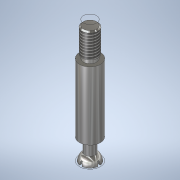
# Autodesk Inventor part: Connecting Pin L24
Saved by Autodesk Inventor 2022 (Build 260153000, 153)
## iProperties
Perskaiciuoti: 1
RuleStatus: InUse
Created: 2009-08-21
Material: Nickel-Copper Alloy 400
Description: Minifix Connecting Pin
Document SubType Name: Modeling
Designer: Saulius Dereskeviciu
Mass: 10.9743 g
Surface Area: 8.70491 cm^2
Volume: 1.24284 cm^3
Density: 8.83 g/cm^3
Appearance: Chrome - Polished
Author: Saulius Dereskeviciu
Part Number: Connecting Pin L24
Autodesk Inventor part; units mm, degrees
ref_plane "YZ Plane" through (0, 0, 0) normal (1, 0, 0) x (0, 1, 0)
ref_plane "XZ Plane" through (0, 0, 0) normal (0, 1, 0) x (-1, 0, 0)
sketch "Sketch1" plane through (0, 0, 0) normal (0, 0, 1) x (1, 0, 0)
  circle A0 centre (0, 0) radius 2
  dimension "d0" = 4
  constraints: 1 centre point, 1 coincident
  measures "d0" diameter of A0
extrude "Extrusion1" add sketch "Sketch1" along normal blind 34
sketch "Sketch2" plane through (0, 0, 0) normal (0, 0, -1) x (-1, 0, 0)
  circle A0 centre (0, 0) radius 2 projected
  circle A1 centre (0, 0) radius 3.5
  line L0 (0, -3.5) -> (0, 3.5)
  dimension "d3" = 7
  constraints: 2 end point, 2 point on circle, 1 centre point, 1 coincident, 1 midpoint, 1 vertical
  measures "d3" diameter of A1
revolve "Revolution1" add sketch "Sketch2" angle 360 about axis through (0, -3.5, 0) along (0, 1, 0) picked at (0.41566, 0.521221) picked at (2.954035, -0.407955) contours A0 L0 | A0 L0 A1
split "Split1" plane through (0, 0, 0) removes the side toward (0, 0, -1)
sketch "Sketch3" plane through (0, 0, 34) normal (0, 0, 1) x (1, 0, 0)
  circle A0 centre (0, 0) radius 2 projected
  circle A1 centre (0, 0) radius 4
  dimension "d5" = 8
  constraints: 1 centre point, 1 coincident
  measures "d5" diameter of A1
ref_plane "Work Plane1" through (0, 0, 8) normal (0, 0, -1) x (-1, 0, 0)
extrude "Extrusion2" add sketch "Sketch3" against normal up to surface (26 mm away)
sketch "Sketch4" plane through (0, 0, 34) normal (0, 0, 1) x (1, 0, 0)
  circle A0 centre (0, 0) radius 4 projected
  circle A1 centre (0, 0) radius 3
  dimension "d9" = 6
  constraints: 1 centre point, 1 coincident
  measures "d9" diameter of A1
extrude "Extrusion3" add sketch "Sketch4" along normal blind 11 contours A1
sketch "Sketch5" plane through (0, 0, 0) normal (0, 1, 0) x (-1, 0, 0)
  line L0 (3, 34) -> (3, 45) projected
  line L1 (-3, 34) -> (3, 34) projected
  line L2 (-4, 34) -> (4, 34) projected
  line L3 (0, -7) -> (0, 42) projected
  line L4 (3, 34) -> (2.5, 34)
  line L5 (2.5, 34) -> (2.5, 35.6)
  line L6 (2.5, 35.6) -> (3, 35.6)
  line L7 (3, 35.6) -> (3, 34)
  point P0 (0, 0)
  dimension "d24" = 1.6
  dimension "d25" = 0.5
  constraints: 8 end point, 2 parallel, 1 collinear, 1 horizontal, 1 perpendicular
  measures "d24" distance of L4.end L5.end
  measures "d25" distance between parallel lines of L0 L5
revolve "Revolution2" cut sketch "Sketch5" angle 360 about axis through (0, 0, -10) along (0, 0, 1)
chamfer "Chamfer1" distance 0.5 angle 45 1 edges at (-3, 0, 45)
thread "Thread1" size "M6x1" class "6g" standard "ISO Metric profile" full length
sketch "Sketch6" plane through (0, 0, 0) normal (0, 0, -1) x (-1, 0, 0)
  circle A0 centre (0, 0) radius 3.5 projected
  line L0 (-0.5, 4) -> (0.5, 4)
  line L1 (0.5, -4) -> (-0.5, -4)
  line L2 (4, 0.5) -> (4, -0.5)
  line L3 (-4, -0.5) -> (-4, 0.5)
  line L4 (-0.5, -4) -> (-0.5, -0.5)
  line L5 (-0.5, 0.5) -> (-0.5, 4)
  line L6 (-4, 0.5) -> (-0.5, 0.5)
  line L7 (0.5, 0.5) -> (4, 0.5)
  line L8 (0.5, 4) -> (0.5, 0.5)
  line L9 (0.5, -0.5) -> (0.5, -4)
  line L10 (4, -0.5) -> (0.5, -0.5)
  line L11 (-0.5, -0.5) -> (-4, -0.5)
  circle A1 centre (0, 0) radius 4 projected
  point P0 (0, 4)
  point P1 (-4, 0)
  dimension "d20" = 1
  constraints: 24 end point, 10 parallel, 8 equal length, 4 perpendicular, 3 horizontal, 2 midpoint, 1 horizontal alignment, 1 tangent, 1 vertical alignment
  measures "d20" distance of L3.start L3.end
sketch "Sketch6 outline for Extrusion4" plane through (0, 0, 0) normal (0, 0, -1) x (-1, 0, 0)
  line L0 (-0.5, 4) -> (0.5, 4)
  line L1 (0.5, 4) -> (0.5, 0.5)
  line L2 (0.5, 0.5) -> (4, 0.5)
  line L3 (4, 0.5) -> (4, -0.5)
  line L4 (4, -0.5) -> (0.5, -0.5)
  line L5 (0.5, -0.5) -> (0.5, -4)
  line L6 (0.5, -4) -> (-0.5, -4)
  line L7 (-0.5, -4) -> (-0.5, -0.5)
  line L8 (-0.5, -0.5) -> (-4, -0.5)
  line L9 (-4, -0.5) -> (-4, 0.5)
  line L10 (-4, 0.5) -> (-0.5, 0.5)
  line L11 (-0.5, 0.5) -> (-0.5, 4)
extrude "Extrusion4" cut sketch "Sketch6 outline for Extrusion4" against normal blind 1.5 draft -10
sketch "Sketch7" plane through (0, 0, 34) normal (0, 0, 1) x (1, 0, 0)
  circle A0 centre (0, 0) radius 4
  dimension "d26" = 8
  constraints: 1 centre point, 1 coincident
  measures "d26" diameter of A0
extrude "Extrusion5" add sketch "Sketch7" against normal blind 34 separate body
sketch "Sketch8" plane through (0, 0, 34) normal (0, 0, 1) x (1, 0, 0)
  circle A0 centre (0, 0) radius 2.5
  dimension "d29" = 5
  constraints: 1 centre point, 1 coincident
  measures "d29" diameter of A0
extrude "Extrusion6" add sketch "Sketch8" along normal blind 13 bodies 2
equation "\"d1\" = Bolt_L"
equation "\"d7\" = Bolt_L"
equation "\"d27\" = Bolt_L"
equation "\"Bolt_L\" = 34"
